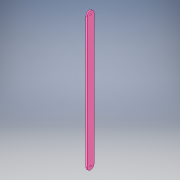
# Autodesk Inventor part: Tie Rod 2
Saved by Autodesk Inventor 2017 (Build 210142000, 142)
## iProperties
Created: 2017-01-25
Part Number: Tie Rod 2
Material: Generic
Document SubType Name: Modeling
Designer: Ben
Density: 1 g/cm^3
Appearance: Pink
Author: Ben
Autodesk Inventor part; units mm, degrees
ref_plane "YZ Plane" through (0, 0, 0) normal (1, 0, 0) x (0, 1, 0)
ref_plane "XZ Plane" through (0, 0, 0) normal (0, 1, 0) x (-1, 0, 0)
ref_plane "XY Plane" through (0, 0, 0) normal (0, 0, 1) x (1, 0, 0)
sketch "Sketch1" plane through (0, 0, 0) normal (1, 0, 0) x (0, 1, 0)
  circle A0 centre (0, 0) radius 1.905
  line L0 (0, 0) -> (356.87, 0) construction
  circle A1 centre (356.87, 0) radius 1.905
  arc A2 (0, 9.525) -> (0, -9.525) centre (0, 0) ccw
  arc A3 (356.87, -9.525) -> (356.87, 9.525) centre (356.87, 0) ccw
  line L1 (356.87, -9.525) -> (0, -9.525)
  line L2 (356.87, 9.525) -> (0, 9.525)
  dimension "d0" = 3.81
  dimension "d1" = 356.87
  dimension "d2" = 19.05
  constraints: 6 end point, 4 centre point, 4 coincident, 4 point on circle, 3 tangent, 2 equal radius, 2 horizontal
  measures "d0" diameter of A0
  measures "d1" distance of L0.start L0.end
  measures "d2" diameter of A3
extrude "Extrusion1" add sketch "Sketch1" along normal blind 3.175
body "Solid1"
